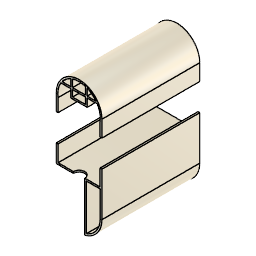
BatteryMounts (Autodesk Fusion 360 design; units mm, degrees)
Autodesk Fusion 360 part; units mm, degrees
note: some values were not read from the file. Set by a fixed rule: which sketch regions a step uses.
sketch "Front" plane through (0, 0, 0) normal (0, 1, 0) x (1, 0, 0)
  circle A0 centre (0, 0) radius 35.56
  line L0 (-123.0104, 0) -> (123.0104, 0) construction
  line L1 (-35.2811, -4.445) -> (35.2811, -4.445)
  line L2 (0, -192.2069) -> (0, 192.2069) construction
  line L3 (-32.639, -3.175) -> (32.639, -3.175)
  line L4 (32.639, -3.175) -> (32.639, 91.44)
  line L5 (32.639, 91.44) -> (-32.639, 91.44)
  line L6 (-32.639, 91.44) -> (-32.639, -3.175)
  line L7 (-32.639, 91.44) -> (32.639, -3.175) construction
  line L8 (-32.639, -3.175) -> (32.639, 91.44) construction
  line L9 (12.7, -4.445) -> (12.7, -17.145)
  circle A1 centre (0, 135.3312) radius 35.56
  line L10 (-118.5711, 135.3312) -> (118.5711, 135.3312) construction
  line L11 (-121.8331, -35.56) -> (121.8331, -35.56) construction
  line L12 (-118.3233, 170.8912) -> (118.3233, 170.8912) construction
  line L13 (-35.56, 92.71) -> (35.56, 92.71)
  line L14 (-35.56, 135.3312) -> (-35.56, 92.71)
  line L15 (35.56, 135.3312) -> (35.56, 92.71)
  line L16 (12.7, -17.145) -> (31.1539, -17.145)
  line L17 (-12.7, -4.445) -> (-12.7, -17.145)
  line L18 (-12.7, -17.145) -> (-31.1539, -17.145)
  line L19 (-35.56, 92.71) -> (-32.639, 92.71)
  line L20 (-32.639, 92.71) -> (-32.639, 67.31)
  line L21 (-32.639, 67.31) -> (-35.56, 67.31)
  line L22 (-35.56, 67.31) -> (-35.56, 92.71)
  line L23 (35.56, 92.71) -> (32.639, 92.71)
  line L24 (32.639, 92.71) -> (32.639, 67.31)
  line L25 (32.639, 67.31) -> (35.56, 67.31)
  line L26 (35.56, 67.31) -> (35.56, 92.71)
  line L27 (-35.56, 95.25) -> (35.56, 95.25)
  circle A2 centre (0, 0) radius 33.02
  circle A3 centre (0, 135.3312) radius 33.02
  line L28 (-26.5108, -19.685) -> (-18.415, -19.685)
  line L29 (18.415, -19.685) -> (26.5108, -19.685)
  line L30 (10.16, -17.145) -> (10.16, -6.985)
  line L31 (10.16, -6.985) -> (-10.16, -6.985)
  line L32 (-10.16, -6.985) -> (-10.16, -17.145)
  line L33 (-18.415, -19.685) -> (18.415, -19.685)
  line L34 (-12.7, -17.145) -> (12.7, -17.145)
  line L35 (-33.02, 95.25) -> (-33.02, 135.3312)
  line L36 (33.02, 95.25) -> (33.02, 135.3312)
  line L37 (8.89, 95.25) -> (8.89, 169.762)
  line L38 (11.43, 95.25) -> (11.43, 169.0042)
  line L39 (-12.7, -17.145) -> (-12.7, -30.48)
  line L40 (-10.16, -17.145) -> (-10.16, -31.4181)
  line L41 (10.16, -17.145) -> (10.16, -31.4181)
  line L42 (12.7, -17.145) -> (12.7, -30.48)
  line L43 (-35.56, 0) -> (-32.639, 0)
  line L44 (-32.639, 0) -> (-32.639, 25.4)
  line L45 (-32.639, 25.4) -> (-35.56, 25.4)
  line L46 (-35.56, 25.4) -> (-35.56, 0)
  line L47 (35.56, 0) -> (32.639, 0)
  line L48 (32.639, 0) -> (32.639, 25.4)
  line L49 (32.639, 25.4) -> (35.56, 25.4)
  line L50 (35.56, 25.4) -> (35.56, 0)
  point P0 (0, 44.1325)
  point P1 (0, -35.56)
  point P2 (0, -12.7)
  point P3 (0, 170.8912)
  point P4 (0, 148.0312)
  dimension "d1" = 71.12
  dimension "d4" = 65.278
  dimension "d5" = 94.615
  dimension "d14" = 71.12
  dimension "d15" = 135.3312
  dimension "d17" = 1.27
  dimension "d23" = 1.27
  dimension "d31" = 31.115
  dimension "d32" = 206.4512
  dimension "d33" = 78.1812
  dimension "d34" = 12.7
  dimension "d35" = 12.7
  dimension "d39" = 12.7
  dimension "d40" = 12.7
  dimension "d45" = 25.4
  dimension "d46" = 25.4
  dimension "d51" = 2.54
  dimension "d56" = 66.04
  dimension "d58" = 66.04
  dimension "d59" = 2.54
  dimension "d60" = 2.54
  dimension "d63" = 2.54
  dimension "d64" = 2.54
  dimension "d66" = 2.54
  dimension "d74" = 2.54
  dimension "d75" = 2.54
  dimension "d79" = 2.54
  dimension "d80" = 44.45
  dimension "d90" = 44.45
  dimension "d92" = 40.0812
  dimension "d102" = 25.4
  dimension "d103" = 25.4
  constraint coincident A0.centre A2.centre
  constraint horizontal L0
  constraint midpoint A0.centre L0
  constraint perpendicular L0 L2
  constraint midpoint A0.centre L2
  constraint horizontal L3
  constraint vertical L4
  constraint horizontal L5
  constraint vertical L6
  constraint midpoint L7 P0
  constraint coincident L2 P0
  constraint coincident L1 L9.start
  constraint perpendicular L1 L9
  constraint coincident L2 A1.centre
  constraint horizontal L10
  constraint midpoint A1.centre L10
  constraint coincident L2 P1
  constraint coincident A0 P1
  constraint horizontal L11
  constraint midpoint P1 L11
  constraint coincident L2 P2
  constraint horizontal L12
  constraint coincident A1 P3
  constraint coincident L2 P3
  constraint midpoint L12 P3
  constraint coincident L2 P4
  constraint parallel L0 L13
  constraint coincident A1 L14.start
  constraint coincident L10 L14.start
  constraint coincident L13 L14.end
  constraint tangent A1 L14
  constraint coincident A1 L15.start
  constraint coincident L10 L15.start
  constraint coincident L13 L15.end
  constraint tangent A1 L15
  constraint coincident A0 L16.end
  constraint perpendicular L9 L16
  constraint coincident L1 L17.start
  constraint perpendicular L1 L17
  constraint coincident A0 L18.end
  constraint perpendicular L17 L18
  constraint horizontal L19
  constraint vertical L20
  constraint horizontal L21
  constraint vertical L22
  constraint horizontal L23
  constraint vertical L24
  constraint horizontal L25
  constraint vertical L26
  constraint coincident L14 L27.start
  constraint coincident L15 L27.end
  constraint perpendicular L15 L27
  constraint concentric A0 A2
  constraint coincident A0 L1.start
  constraint coincident A0 L1.end
  constraint concentric A1 A3
  constraint coincident A2 L28.start
  constraint parallel L18 L28
  constraint coincident A2 L29.end
  constraint vertical L30
  constraint horizontal L31
  constraint vertical L32
  constraint coincident L32.end L34
  constraint coincident L30.start L34
  constraint coincident L27 L35.start
  constraint perpendicular L27 L35
  constraint coincident L27 L36.start
  constraint perpendicular L27 L36
  constraint coincident A3 L35.end
  constraint coincident L10 L35.end
  constraint coincident A3 L36.end
  constraint coincident L10 L36.end
  constraint coincident L27 L37.start
  constraint perpendicular L10 L37
  constraint coincident L27 L38.start
  constraint perpendicular L10 L38
  constraint coincident A1 L37.end
  constraint coincident A1 L38.end
  constraint coincident A2 L39.end
  constraint perpendicular L33 L39
  constraint coincident A2 L40.end
  constraint perpendicular L34 L40
  constraint coincident A2 L41.end
  constraint perpendicular L34 L41
  constraint coincident A2 L42.end
  constraint perpendicular L34 L42
  constraint coincident L6 L20.end
  constraint coincident L4 L24.end
  constraint horizontal L43
  constraint vertical L44
  constraint horizontal L45
  constraint vertical L46
  constraint coincident A0 L43.start
  constraint coincident L0 L43.start
  constraint horizontal L47
  constraint vertical L48
  constraint horizontal L49
  constraint vertical L50
  constraint coincident L0 L47.start
  constraint coincident A0 L47.start
  constraint coincident L6 L44.end
  constraint coincident L4 L48.end
  measures "d1" diameter of A0
  measures "d4" distance of L4.end L5.end
  measures "d5" distance of L3.start L5.end
  measures "d14" diameter of A1
  measures "d15" distance of A0.centre A1.centre
  measures "d17" distance of L1 L3
  measures "d23" distance of L5 L13
  measures "d31" distance of L1 L11
  measures "d32" distance of L11 L12
  measures "d33" distance of L12 L13
  measures "d34" distance of L17.start L17.end
  measures "d35" distance of L9.start L9.end
  measures "d39" distance of L2 L17
  measures "d40" distance of L2 L9
  measures "d45" distance of L13.start L21.end
  measures "d46" distance of L13.end L25.end
  measures "d51" distance of L13 L27
  measures "d56" diameter of A2
  measures "d58" diameter of A3
  measures "d59" distance of L18 L28
  measures "d60" distance of L16 L29
  measures "d63" distance of L17 L32
  measures "d64" distance of L9 L30
  measures "d66" distance of L1 L31
  measures "d74" distance of L14 L35
  measures "d75" distance of L15 L36
  measures "d79" distance of L37 L38
  measures "d80" distance of L14 L37
  measures "d90" distance of L14 L37
  measures "d92" distance of L10 L27
  measures "d102" distance of L43.start L45.end
  measures "d103" distance of L47.start L49.end
extrude "Extrude1" add sketch "Front" along normal blind 152.4 contours A0 L1 A2 L43 | A0 L6 L44 L45 L46 | A0 L6 A2 L43 L44 | A0 L1 L18 A2 | A0 L16 L18 A2 | A0 L4 L48 L49 L50 | A0 L4 A2 L47 L48 | A0 L1 L16 A2 | L18 A2 L28 L33 L39 | L1 L9 L17 L30 L31 L32 L34 | A0 L1 A2 L47 | L16 A2 L29 L33 L42 | L33 L34 L39 L40 | L33 L34 L41 L42 | L33 L34 L40 L41 | A2 L33 L39 L40 | A2 L33 L41 L42 makes body 1
extrude "Extrude9" add sketch "Front" along normal blind 152.4 separate body contours L6 L13 L19 L20 L21 L22 | L4 L13 L23 L24 L25 L26 | L13 L14 L15 L19 L23 L27 | A1 L14 L27 L35 | A1 L15 L27 L36 | A1 A3 L35 L37 | A1 A3 L36 L38 | A1 A3 L37 L38 picked at (5.7285, 169.4993) picked at (12.9397, 167.4743) picked at (9.4589, 167.8477) makes body 2
extrude "Extrude10" add sketch "Front" along normal blind 82.55 contours A1 A3 L37 L38 | A1 L27 L37 L38 | A3 L37 L38 | A1 A3 L37 L38 bodies 2
sketch "Motor Cut-out" plane through (-35.56, 0, 0) normal (-1, 0, 0) x (0, -1, 0)
  line L0 (0, -135.3312) -> (0, -67.31)
  line L1 (0, -67.31) -> (-152.4, -67.31)
  line L2 (-152.4, -67.31) -> (-152.4, -135.3312)
  line L3 (-152.4, -135.3312) -> (0, -135.3312)
  line L4 (0, -95.25) -> (-82.55, -95.25)
  line L5 (-82.55, -95.25) -> (-82.55, -172.55)
  line L6 (-82.55, -172.55) -> (0, -172.55)
  line L7 (0, -172.55) -> (0, -95.25)
  dimension "d86" = 82.55
  dimension "d91" = 40.0812
  constraint horizontal L4
  constraint vertical L5
  constraint horizontal L6
  constraint vertical L7
  constraint coincident L0 L4.start
  measures "d86" distance of L4.start L4.end
  measures "d91" distance of L3 L4
extrude "Extrude11" cut sketch "Motor Cut-out" against normal blind 44.45 contours L0 L3 L4 L5 L7 | L3 L5 L6 L7 bodies 2
sketch "3d-Print Arch" plane through (8.89, 0, 0) normal (-1, 0, 0) x (0, -1, 0)
  line L0 (0, -169.762) -> (0, -95.25)
  line L1 (0, -95.25) -> (-82.55, -95.25)
  line L2 (-82.55, -95.25) -> (-82.55, -167.132)
  line L3 (-82.55, -167.132) -> (-82.55, -169.762)
  line L4 (-82.55, -169.762) -> (0, -169.762)
  line L5 (-82.55, -95.25) -> (-82.55, -167.132) construction
  line L6 (-104.9543, -131.191) -> (-60.1457, -131.191) construction
  circle A0 centre (-87.63, -131.191) radius 35.941
  point P0 (-82.55, -131.191)
  dimension "d98" = 71.882
  dimension "d100" = 71.882
  dimension "d101" = 5.08
  constraint coincident L1.end L2.start
  constraint coincident L2.end L3.start
  constraint midpoint L5 P0
  constraint horizontal L6
  constraint coincident L6 A0.centre
  measures "d98" distance of L1.end L2.end
  measures "d100" diameter of A0
  measures "d101" distance of P0 A0.centre
extrude "Extrude12" cut sketch "3d-Print Arch" against normal blind 2.54 contours L2 A0 picked at (-66.6022, -131.7672) bodies 2
sketch "Sketch8" plane through (0, 0, -92.71) normal (0, 0, 1) x (-1, 0, 0)
  line L0 (32.639, 0) -> (-32.639, 0)
  line L1 (-32.639, 0) -> (-32.639, -152.4)
  line L2 (-32.639, -152.4) -> (32.639, -152.4)
  line L3 (32.639, -152.4) -> (32.639, 0)
  circle A0 centre (0, 0) radius 8.89
  dimension "d104" = 17.78
  constraint coincident A0.centre origin
  measures "d104" diameter of A0
extrude "Extrude13" cut sketch "Sketch8" against normal blind 12.7 contours L0 A0 picked at (-0.6008, -4.8695) bodies 2
equation "d1 = ( ( 1.5 * 2 ) * 1 in ) - ( ( 0.1 * 2 ) * 1 in )"
equation "d6 = ( ( 2.80 - 1 ) / 2 ) * 1 in"
equation "d10 = ( d1 - d4 - 0.1 in ) / 2"
equation "d14 = d1"
equation "d17 = d23"
equation "d33 = 2.75 in + 0.328 in"
equation "d35 = d34"
equation "d46 = d45"
equation "d56 = d1 - ( ( 0.1 * 2 ) * 1 in )"
equation "d58 = d1 - ( ( 0.1 * 2 ) * 1 in )"
equation "d83 = 6 in - 2.75 in"
equation "d86 = 6 in - 2.75 in"
equation "d97 = ( ( 2.9335441712 / 2 ) * 1 in ) - 0.1 in"
equation "d102 = d45"
equation "d103 = d45"
named bodies: "Top", "Bottom"
